Autodesk Fusion 360 part; units mm, degrees
(part 4 of 11)
  spline S51 degree 5 poles (-18.4507, -20.1557) (-18.4538, -20.1562) (-18.4598, -20.1573) (-18.469, -20.1589) (-18.4811, -20.161) (-18.4962, -20.1638) (-18.5113, -20.1666) (-18.5264, -20.1695) (-18.5414, -20.1724) (-18.5564, -20.1754) (-18.5713, -20.1785) (-18.5862, -20.1816) (-18.6011, -20.1848) (-18.6159, -20.1881) (-18.6307, -20.1914) (-18.6455, -20.1948) (-18.6602, -20.1983) (-18.6749, -20.2018) (-18.6895, -20.2054) (-18.7041, -20.209) (-18.7186, -20.2127) (-18.7332, -20.2165) (-18.7476, -20.2203) (-18.762, -20.2242) (-18.7764, -20.2282) (-18.7908, -20.2323) (-18.805, -20.2364) (-18.8193, -20.2406) (-18.8335, -20.2448) (-18.8476, -20.2491) (-18.8617, -20.2535) (-18.8758, -20.2579) (-18.8898, -20.2625) (-18.9038, -20.267) (-18.9177, -20.2717) (-18.9315, -20.2764) (-18.9453, -20.2812) (-18.9591, -20.2861) (-18.9728, -20.2911) (-18.9865, -20.2961) (-19.0001, -20.3012) (-19.0136, -20.3063) (-19.0271, -20.3116) (-19.0405, -20.3169) (-19.0539, -20.3223) (-19.0672, -20.3278) (-19.0805, -20.3333) (-19.0937, -20.3389) (-19.1068, -20.3447) (-19.1199, -20.3504) (-19.1329, -20.3563) (-19.1458, -20.3623) (-19.1587, -20.3683) (-19.1715, -20.3745) (-19.1842, -20.3807) (-19.1968, -20.387) (-19.2094, -20.3934) (-19.2219, -20.3999) (-19.2344, -20.4065) (-19.2468, -20.4131) (-19.259, -20.4199) (-19.2712, -20.4268) (-19.2832, -20.4339) (-19.2952, -20.4411) (-19.307, -20.4484) (-19.3187, -20.4558) (-19.3304, -20.4633) (-19.342, -20.4709) (-19.3535, -20.4785) (-19.3649, -20.4864) (-19.376, -20.4945) (-19.3846, -20.5013) (-19.3909, -20.5066) (-19.395, -20.5103) (-19.397, -20.5122) knots -1 -1 -1 -1 -1 -1 -0.98571429 -0.97142857 -0.95714286 -0.94285714 -0.92857143 -0.91428571 -0.9 -0.88571429 -0.87142857 -0.85714286 -0.84285714 -0.82857143 -0.81428571 -0.8 -0.78571429 -0.77142857 -0.75714286 -0.74285714 -0.72857143 -0.71428571 -0.7 -0.68571429 -0.67142857 -0.65714286 -0.64285714 -0.62857143 -0.61428571 -0.6 -0.58571429 -0.57142857 -0.55714286 -0.54285714 -0.52857143 -0.51428571 -0.5 -0.48571429 -0.47142857 -0.45714286 -0.44285714 -0.42857143 -0.41428571 -0.4 -0.38571429 -0.37142857 -0.35714286 -0.34285714 -0.32857143 -0.31428571 -0.3 -0.28571429 -0.27142857 -0.25714286 -0.24285714 -0.22857143 -0.21428571 -0.2 -0.18571429 -0.17142857 -0.15714286 -0.14285714 -0.12857143 -0.11428571 -0.1 -0.08571429 -0.07142857 -0.05714286 -0.04285714 -0.02857143 -0.01428571 0 0 0 0 0 0 construction
  line L57 (-19.397, -20.5122) -> (-19.4476, -20.5584) construction
  arc A104 (-19.7933, -20.5503) -> (-19.4476, -20.5584) centre (-19.6162, -20.3738) ccw construction
  arc A105 (-19.7933, -20.5503) -> (-19.8754, -20.4695) centre (-23.9648, -24.7074) ccw construction
  arc A106 (-19.8891, -20.1239) -> (-19.8754, -20.4695) centre (-19.7018, -20.2896) ccw construction
  line L58 (-19.8891, -20.1239) -> (-19.8437, -20.0726) construction
  spline S52 degree 5 poles (-19.8437, -20.0726) (-19.8419, -20.0705) (-19.8383, -20.0664) (-19.8331, -20.06) (-19.8264, -20.0513) (-19.8184, -20.0401) (-19.8108, -20.0286) (-19.8033, -20.017) (-19.7959, -20.0052) (-19.7887, -19.9934) (-19.7814, -19.9816) (-19.7743, -19.9696) (-19.7673, -19.9576) (-19.7604, -19.9454) (-19.7537, -19.9332) (-19.7471, -19.9208) (-19.7406, -19.9083) (-19.7343, -19.8958) (-19.728, -19.8831) (-19.7218, -19.8704) (-19.7157, -19.8577) (-19.7097, -19.8449) (-19.7037, -19.832) (-19.6979, -19.819) (-19.6921, -19.806) (-19.6865, -19.7929) (-19.6809, -19.7797) (-19.6754, -19.7665) (-19.67, -19.7532) (-19.6647, -19.7399) (-19.6594, -19.7265) (-19.6542, -19.713) (-19.6491, -19.6995) (-19.6441, -19.6859) (-19.6391, -19.6723) (-19.6343, -19.6586) (-19.6295, -19.6449) (-19.6247, -19.6311) (-19.6201, -19.6173) (-19.6155, -19.6034) (-19.611, -19.5895) (-19.6066, -19.5755) (-19.6022, -19.5614) (-19.5979, -19.5474) (-19.5937, -19.5332) (-19.5895, -19.5191) (-19.5855, -19.5048) (-19.5814, -19.4906) (-19.5775, -19.4763) (-19.5736, -19.4619) (-19.5698, -19.4475) (-19.5661, -19.4331) (-19.5624, -19.4186) (-19.5588, -19.4041) (-19.5552, -19.3895) (-19.5518, -19.3749) (-19.5483, -19.3603) (-19.545, -19.3456) (-19.5417, -19.3308) (-19.5385, -19.3161) (-19.5354, -19.3013) (-19.5323, -19.2864) (-19.5293, -19.2715) (-19.5263, -19.2566) (-19.5234, -19.2417) (-19.5206, -19.2267) (-19.5178, -19.2116) (-19.5151, -19.1966) (-19.5125, -19.1815) (-19.5099, -19.1663) (-19.5074, -19.1512) (-19.5054, -19.139) (-19.504, -19.1298) (-19.503, -19.1237) (-19.5026, -19.1207) knots 0 0 0 0 0 0 0.01428571 0.02857143 0.04285714 0.05714286 0.07142857 0.08571429 0.1 0.11428571 0.12857143 0.14285714 0.15714286 0.17142857 0.18571429 0.2 0.21428571 0.22857143 0.24285714 0.25714286 0.27142857 0.28571429 0.3 0.31428571 0.32857143 0.34285714 0.35714286 0.37142857 0.38571429 0.4 0.41428571 0.42857143 0.44285714 0.45714286 0.47142857 0.48571429 0.5 0.51428571 0.52857143 0.54285714 0.55714286 0.57142857 0.58571429 0.6 0.61428571 0.62857143 0.64285714 0.65714286 0.67142857 0.68571429 0.7 0.71428571 0.72857143 0.74285714 0.75714286 0.77142857 0.78571429 0.8 0.81428571 0.82857143 0.84285714 0.85714286 0.87142857 0.88571429 0.9 0.91428571 0.92857143 0.94285714 0.95714286 0.97142857 0.98571429 1 1 1 1 1 1 construction
  arc A107 (-19.5026, -19.1207) -> (-19.8167, -18.8837) centre (-23.9648, -24.7074) ccw construction
  spline S53 degree 5 poles (-19.8167, -18.8837) (-19.8195, -18.885) (-19.8251, -18.8875) (-19.8335, -18.8914) (-19.8446, -18.8967) (-19.8585, -18.9032) (-19.8724, -18.9099) (-19.8862, -18.9166) (-19.8999, -18.9233) (-19.9136, -18.9301) (-19.9273, -18.9369) (-19.9409, -18.9438) (-19.9544, -18.9507) (-19.9679, -18.9577) (-19.9813, -18.9647) (-19.9947, -18.9718) (-20.008, -18.979) (-20.0213, -18.9862) (-20.0345, -18.9934) (-20.0476, -19.0007) (-20.0607, -19.0081) (-20.0738, -19.0155) (-20.0867, -19.0229) (-20.0996, -19.0304) (-20.1125, -19.038) (-20.1253, -19.0456) (-20.138, -19.0533) (-20.1507, -19.061) (-20.1633, -19.0688) (-20.1759, -19.0766) (-20.1884, -19.0845) (-20.2008, -19.0924) (-20.2132, -19.1004) (-20.2255, -19.1085) (-20.2377, -19.1166) (-20.2499, -19.1247) (-20.2619, -19.1329) (-20.274, -19.1412) (-20.2859, -19.1495) (-20.2978, -19.1579) (-20.3096, -19.1663) (-20.3214, -19.1748) (-20.3331, -19.1834) (-20.3447, -19.192) (-20.3562, -19.2007) (-20.3676, -19.2094) (-20.379, -19.2182) (-20.3903, -19.2271) (-20.4015, -19.236) (-20.4126, -19.2449) (-20.4237, -19.254) (-20.4346, -19.2631) (-20.4455, -19.2723) (-20.4562, -19.2815) (-20.4669, -19.2908) (-20.4775, -19.3002) (-20.488, -19.3096) (-20.4984, -19.3191) (-20.5087, -19.3287) (-20.519, -19.3384) (-20.5291, -19.3481) (-20.539, -19.3579) (-20.5488, -19.3678) (-20.5585, -19.3779) (-20.568, -19.388) (-20.5774, -19.3982) (-20.5868, -19.4085) (-20.596, -19.4188) (-20.6052, -19.4291) (-20.6141, -19.4397) (-20.6227, -19.4504) (-20.6293, -19.4592) (-20.634, -19.466) (-20.637, -19.4706) (-20.6385, -19.4729) knots -1 -1 -1 -1 -1 -1 -0.98571429 -0.97142857 -0.95714286 -0.94285714 -0.92857143 -0.91428571 -0.9 -0.88571429 -0.87142857 -0.85714286 -0.84285714 -0.82857143 -0.81428571 -0.8 -0.78571429 -0.77142857 -0.75714286 -0.74285714 -0.72857143 -0.71428571 -0.7 -0.68571429 -0.67142857 -0.65714286 -0.64285714 -0.62857143 -0.61428571 -0.6 -0.58571429 -0.57142857 -0.55714286 -0.54285714 -0.52857143 -0.51428571 -0.5 -0.48571429 -0.47142857 -0.45714286 -0.44285714 -0.42857143 -0.41428571 -0.4 -0.38571429 -0.37142857 -0.35714286 -0.34285714 -0.32857143 -0.31428571 -0.3 -0.28571429 -0.27142857 -0.25714286 -0.24285714 -0.22857143 -0.21428571 -0.2 -0.18571429 -0.17142857 -0.15714286 -0.14285714 -0.12857143 -0.11428571 -0.1 -0.08571429 -0.07142857 -0.05714286 -0.04285714 -0.02857143 -0.01428571 0 0 0 0 0 0 construction
  line L59 (-20.6385, -19.4729) -> (-20.6753, -19.5306) construction
  arc A108 (-21.0114, -19.6123) -> (-20.6753, -19.5306) centre (-20.886, -19.396) ccw construction
  arc A109 (-21.0114, -19.6123) -> (-21.1116, -19.5555) centre (-23.9648, -24.7074) ccw construction
  arc A110 (-21.2143, -19.2252) -> (-21.1116, -19.5555) centre (-20.9905, -19.3368) ccw construction
  line L60 (-21.2143, -19.2252) -> (-21.1837, -19.1639) construction
  spline S54 degree 5 poles (-21.1837, -19.1639) (-21.1825, -19.1615) (-21.1801, -19.1565) (-21.1767, -19.149) (-21.1725, -19.1389) (-21.1677, -19.126) (-21.1633, -19.1129) (-21.1591, -19.0997) (-21.155, -19.0865) (-21.151, -19.0732) (-21.1471, -19.0599) (-21.1433, -19.0465) (-21.1397, -19.033) (-21.1362, -19.0195) (-21.1329, -19.0059) (-21.1297, -18.9923) (-21.1267, -18.9786) (-21.1238, -18.9648) (-21.121, -18.951) (-21.1183, -18.9371) (-21.1157, -18.9232) (-21.1132, -18.9093) (-21.1108, -18.8953) (-21.1085, -18.8812) (-21.1063, -18.8672) (-21.1042, -18.853) (-21.1022, -18.8389) (-21.1004, -18.8247) (-21.0986, -18.8105) (-21.0969, -18.7962) (-21.0953, -18.7819) (-21.0937, -18.7675) (-21.0923, -18.7532) (-21.091, -18.7388) (-21.0897, -18.7243) (-21.0885, -18.7098) (-21.0875, -18.6953) (-21.0865, -18.6808) (-21.0856, -18.6662) (-21.0847, -18.6516) (-21.084, -18.637) (-21.0833, -18.6224) (-21.0827, -18.6077) (-21.0822, -18.593) (-21.0818, -18.5782) (-21.0815, -18.5635) (-21.0812, -18.5487) (-21.081, -18.5339) (-21.0809, -18.519) (-21.0809, -18.5041) (-21.0809, -18.4892) (-21.081, -18.4743) (-21.0812, -18.4594) (-21.0815, -18.4444) (-21.0819, -18.4294) (-21.0823, -18.4144) (-21.0828, -18.3994) (-21.0833, -18.3843) (-21.084, -18.3693) (-21.0847, -18.3542) (-21.0855, -18.3391) (-21.0864, -18.3239) (-21.0873, -18.3088) (-21.0883, -18.2936) (-21.0894, -18.2784) (-21.0905, -18.2632) (-21.0917, -18.2479) (-21.093, -18.2327) (-21.0944, -18.2174) (-21.0958, -18.2021) (-21.0973, -18.1868) (-21.0986, -18.1746) (-21.0996, -18.1654) (-21.1002, -18.1592) (-21.1006, -18.1562) knots 0 0 0 0 0 0 0.01428571 0.02857143 0.04285714 0.05714286 0.07142857 0.08571429 0.1 0.11428571 0.12857143 0.14285714 0.15714286 0.17142857 0.18571429 0.2 0.21428571 0.22857143 0.24285714 0.25714286 0.27142857 0.28571429 0.3 0.31428571 0.32857143 0.34285714 0.35714286 0.37142857 0.38571429 0.4 0.41428571 0.42857143 0.44285714 0.45714286 0.47142857 0.48571429 0.5 0.51428571 0.52857143 0.54285714 0.55714286 0.57142857 0.58571429 0.6 0.61428571 0.62857143 0.64285714 0.65714286 0.67142857 0.68571429 0.7 0.71428571 0.72857143 0.74285714 0.75714286 0.77142857 0.78571429 0.8 0.81428571 0.82857143 0.84285714 0.85714286 0.87142857 0.88571429 0.9 0.91428571 0.92857143 0.94285714 0.95714286 0.97142857 0.98571429 1 1 1 1 1 1 construction
  arc A111 (-21.1006, -18.1562) -> (-21.4653, -18.0085) centre (-23.9648, -24.7074) ccw construction
  spline S55 degree 5 poles (-21.4653, -18.0085) (-21.4677, -18.0105) (-21.4724, -18.0144) (-21.4795, -18.0204) (-21.489, -18.0283) (-21.5007, -18.0382) (-21.5123, -18.0482) (-21.5239, -18.0583) (-21.5355, -18.0683) (-21.547, -18.0784) (-21.5584, -18.0885) (-21.5697, -18.0987) (-21.581, -18.1089) (-21.5922, -18.1192) (-21.6034, -18.1294) (-21.6144, -18.1397) (-21.6255, -18.1501) (-21.6364, -18.1605) (-21.6473, -18.1709) (-21.6581, -18.1813) (-21.6688, -18.1918) (-21.6795, -18.2024) (-21.6901, -18.2129) (-21.7006, -18.2235) (-21.7111, -18.2341) (-21.7215, -18.2448) (-21.7318, -18.2555) (-21.7421, -18.2663) (-21.7522, -18.277) (-21.7623, -18.2878) (-21.7724, -18.2987) (-21.7823, -18.3096) (-21.7922, -18.3205) (-21.802, -18.3314) (-21.8117, -18.3424) (-21.8213, -18.3535) (-21.8309, -18.3645) (-21.8404, -18.3756) (-21.8498, -18.3868) (-21.8591, -18.3979) (-21.8683, -18.4091) (-21.8775, -18.4204) (-21.8865, -18.4317) (-21.8955, -18.443) (-21.9044, -18.4543) (-21.9132, -18.4657) (-21.9219, -18.4772) (-21.9305, -18.4887) (-21.939, -18.5002) (-21.9474, -18.5117) (-21.9558, -18.5233) (-21.964, -18.5349) (-21.9721, -18.5466) (-21.9801, -18.5583) (-21.988, -18.5701) (-21.9958, -18.5819) (-22.0035, -18.5937) (-22.0111, -18.6056) (-22.0186, -18.6175) (-22.026, -18.6295) (-22.0332, -18.6415) (-22.0403, -18.6535) (-22.0472, -18.6657) (-22.0539, -18.6779) (-22.0605, -18.6901) (-22.067, -18.7024) (-22.0733, -18.7147) (-22.0796, -18.7271) (-22.0858, -18.7395) (-22.0917, -18.7519) (-22.0972, -18.7645) (-22.1013, -18.7747) (-22.104, -18.7825) (-22.1058, -18.7877) (-22.1066, -18.7903) knots -1 -1 -1 -1 -1 -1 -0.98571429 -0.97142857 -0.95714286 -0.94285714 -0.92857143 -0.91428571 -0.9 -0.88571429 -0.87142857 -0.85714286 -0.84285714 -0.82857143 -0.81428571 -0.8 -0.78571429 -0.77142857 -0.75714286 -0.74285714 -0.72857143 -0.71428571 -0.7 -0.68571429 -0.67142857 -0.65714286 -0.64285714 -0.62857143 -0.61428571 -0.6 -0.58571429 -0.57142857 -0.55714286 -0.54285714 -0.52857143 -0.51428571 -0.5 -0.48571429 -0.47142857 -0.45714286 -0.44285714 -0.42857143 -0.41428571 -0.4 -0.38571429 -0.37142857 -0.35714286 -0.34285714 -0.32857143 -0.31428571 -0.3 -0.28571429 -0.27142857 -0.25714286 -0.24285714 -0.22857143 -0.21428571 -0.2 -0.18571429 -0.17142857 -0.15714286 -0.14285714 -0.12857143 -0.11428571 -0.1 -0.08571429 -0.07142857 -0.05714286 -0.04285714 -0.02857143 -0.01428571 0 0 0 0 0 0 construction
  line L61 (-22.1066, -18.7903) -> (-22.1273, -18.8556) construction
  arc A112 (-22.4307, -19.0215) -> (-22.1273, -18.8556) centre (-22.3656, -18.7801) ccw construction
  arc A113 (-22.4307, -19.0215) -> (-22.5423, -18.9926) centre (-23.9648, -24.7074) ccw construction
  arc A114 (-22.7269, -18.7001) -> (-22.5423, -18.9926) centre (-22.4819, -18.75) ccw construction
  line L62 (-22.7269, -18.7001) -> (-22.7132, -18.633) construction
  spline S56 degree 5 poles (-22.7132, -18.633) (-22.7127, -18.6303) (-22.7116, -18.6249) (-22.7103, -18.6168) (-22.7089, -18.6059) (-22.7076, -18.5922) (-22.7067, -18.5784) (-22.7061, -18.5646) (-22.7056, -18.5508) (-22.7051, -18.5369) (-22.7048, -18.523) (-22.7046, -18.5091) (-22.7046, -18.4952) (-22.7047, -18.4812) (-22.705, -18.4673) (-22.7055, -18.4532) (-22.7061, -18.4392) (-22.7069, -18.4252) (-22.7078, -18.4111) (-22.7087, -18.397) (-22.7098, -18.3829) (-22.711, -18.3688) (-22.7123, -18.3546) (-22.7137, -18.3405) (-22.7153, -18.3263) (-22.7169, -18.3122) (-22.7187, -18.298) (-22.7205, -18.2838) (-22.7225, -18.2696) (-22.7245, -18.2553) (-22.7267, -18.2411) (-22.7289, -18.2269) (-22.7312, -18.2126) (-22.7337, -18.1983) (-22.7362, -18.1841) (-22.7388, -18.1698) (-22.7415, -18.1555) (-22.7443, -18.1412) (-22.7472, -18.1269) (-22.7502, -18.1126) (-22.7533, -18.0983) (-22.7564, -18.0839) (-22.7597, -18.0696) (-22.763, -18.0553) (-22.7664, -18.0409) (-22.7699, -18.0266) (-22.7735, -18.0122) (-22.7771, -17.9978) (-22.7808, -17.9835) (-22.7847, -17.9691) (-22.7886, -17.9547) (-22.7925, -17.9404) (-22.7966, -17.926) (-22.8007, -17.9116) (-22.8049, -17.8972) (-22.8092, -17.8828) (-22.8136, -17.8684) (-22.8181, -17.854) (-22.8226, -17.8396) (-22.8272, -17.8252) (-22.8319, -17.8108) (-22.8366, -17.7964) (-22.8414, -17.782) (-22.8463, -17.7676) (-22.8513, -17.7532) (-22.8563, -17.7389) (-22.8615, -17.7245) (-22.8667, -17.7101) (-22.8719, -17.6957) (-22.8773, -17.6813) (-22.8827, -17.6669) (-22.8871, -17.6553) (-22.8904, -17.6467) (-22.8926, -17.6409) (-22.8937, -17.6381) knots 0 0 0 0 0 0 0.01428571 0.02857143 0.04285714 0.05714286 0.07142857 0.08571429 0.1 0.11428571 0.12857143 0.14285714 0.15714286 0.17142857 0.18571429 0.2 0.21428571 0.22857143 0.24285714 0.25714286 0.27142857 0.28571429 0.3 0.31428571 0.32857143 0.34285714 0.35714286 0.37142857 0.38571429 0.4 0.41428571 0.42857143 0.44285714 0.45714286 0.47142857 0.48571429 0.5 0.51428571 0.52857143 0.54285714 0.55714286 0.57142857 0.58571429 0.6 0.61428571 0.62857143 0.64285714 0.65714286 0.67142857 0.68571429 0.7 0.71428571 0.72857143 0.74285714 0.75714286 0.77142857 0.78571429 0.8 0.81428571 0.82857143 0.84285714 0.85714286 0.87142857 0.88571429 0.9 0.91428571 0.92857143 0.94285714 0.95714286 0.97142857 0.98571429 1 1 1 1 1 1 construction
  arc A115 (-22.8937, -17.6381) -> (-23.2843, -17.5899) centre (-23.9648, -24.7074) ccw construction
  spline S57 degree 5 poles (-23.2843, -17.5899) (-23.2861, -17.5924) (-23.2896, -17.5974) (-23.2949, -17.605) (-23.302, -17.6151) (-23.3107, -17.6277) (-23.3194, -17.6404) (-23.328, -17.6531) (-23.3366, -17.6658) (-23.345, -17.6785) (-23.3534, -17.6913) (-23.3618, -17.704) (-23.37, -17.7168) (-23.3782, -17.7296) (-23.3863, -17.7424) (-23.3944, -17.7552) (-23.4023, -17.7681) (-23.4102, -17.7809) (-23.418, -17.7938) (-23.4258, -17.8067) (-23.4334, -17.8196) (-23.441, -17.8325) (-23.4485, -17.8455) (-23.456, -17.8584) (-23.4633, -17.8714) (-23.4706, -17.8844) (-23.4778, -17.8974) (-23.4849, -17.9105) (-23.4919, -17.9235) (-23.4989, -17.9366) (-23.5058, -17.9496) (-23.5126, -17.9627) (-23.5193, -17.9758) (-23.5259, -17.9889) (-23.5324, -18.0021) (-23.5389, -18.0152) (-23.5453, -18.0284) (-23.5515, -18.0415) (-23.5577, -18.0547) (-23.5638, -18.0679) (-23.5699, -18.0811) (-23.5758, -18.0944) (-23.5816, -18.1076) (-23.5873, -18.1209) (-23.593, -18.1341) (-23.5985, -18.1474) (-23.604, -18.1607) (-23.6093, -18.174) (-23.6146, -18.1874) (-23.6197, -18.2007) (-23.6248, -18.214) (-23.6297, -18.2274) (-23.6345, -18.2408) (-23.6392, -18.2542) (-23.6438, -18.2676) (-23.6483, -18.281) (-23.6527, -18.2944) (-23.6569, -18.3079) (-23.6611, -18.3213) (-23.6651, -18.3348) (-23.669, -18.3482) (-23.6727, -18.3617) (-23.6762, -18.3752) (-23.6796, -18.3888) (-23.6828, -18.4023) (-23.6858, -18.4158) (-23.6888, -18.4294) (-23.6917, -18.4429) (-23.6944, -18.4565) (-23.6969, -18.4701) (-23.699, -18.4837) (-23.7002, -18.4946) (-23.7009, -18.5028) (-23.7012, -18.5083) (-23.7014, -18.511) knots -1 -1 -1 -1 -1 -1 -0.98571429 -0.97142857 -0.95714286 -0.94285714 -0.92857143 -0.91428571 -0.9 -0.88571429 -0.87142857 -0.85714286 -0.84285714 -0.82857143 -0.81428571 -0.8 -0.78571429 -0.77142857 -0.75714286 -0.74285714 -0.72857143 -0.71428571 -0.7 -0.68571429 -0.67142857 -0.65714286 -0.64285714 -0.62857143 -0.61428571 -0.6 -0.58571429 -0.57142857 -0.55714286 -0.54285714 -0.52857143 -0.51428571 -0.5 -0.48571429 -0.47142857 -0.45714286 -0.44285714 -0.42857143 -0.41428571 -0.4 -0.38571429 -0.37142857 -0.35714286 -0.34285714 -0.32857143 -0.31428571 -0.3 -0.28571429 -0.27142857 -0.25714286 -0.24285714 -0.22857143 -0.21428571 -0.2 -0.18571429 -0.17142857 -0.15714286 -0.14285714 -0.12857143 -0.11428571 -0.1 -0.08571429 -0.07142857 -0.05714286 -0.04285714 -0.02857143 -0.01428571 0 0 0 0 0 0 construction
  line L63 (-23.7014, -18.511) -> (-23.7044, -18.5794) construction
  arc A116 (-23.9546, -18.8182) -> (-23.7044, -18.5794) centre (-23.9542, -18.5682) ccw construction
  arc A117 (-23.9546, -18.8182) -> (-24.0699, -18.8191) centre (-23.9648, -24.7074) ccw construction
  arc A118 (-24.3238, -18.5844) -> (-24.0699, -18.8191) centre (-24.0743, -18.5692) ccw construction
  line L64 (-24.3238, -18.5844) -> (-24.328, -18.5161) construction
  spline S58 degree 5 poles (-24.328, -18.5161) (-24.3282, -18.5133) (-24.3286, -18.5079) (-24.3294, -18.4997) (-24.3308, -18.4888) (-24.3332, -18.4752) (-24.3359, -18.4617) (-24.3388, -18.4482) (-24.3419, -18.4347) (-24.3451, -18.4212) (-24.3484, -18.4077) (-24.3518, -18.3942) (-24.3553, -18.3807) (-24.3591, -18.3673) (-24.363, -18.3538) (-24.3671, -18.3404) (-24.3713, -18.327) (-24.3757, -18.3137) (-24.3802, -18.3003) (-24.3848, -18.2869) (-24.3895, -18.2736) (-24.3943, -18.2603) (-24.3992, -18.247) (-24.4042, -18.2337) (-24.4094, -18.2204) (-24.4146, -18.2071) (-24.42, -18.1939) (-24.4255, -18.1806) (-24.431, -18.1674) (-24.4367, -18.1542) (-24.4425, -18.141) (-24.4483, -18.1278) (-24.4543, -18.1147) (-24.4603, -18.1015) (-24.4664, -18.0884) (-24.4727, -18.0753) (-24.479, -18.0621) (-24.4854, -18.0491) (-24.4919, -18.036) (-24.4985, -18.0229) (-24.5051, -18.0099) (-24.5119, -17.9969) (-24.5187, -17.9839) (-24.5256, -17.9709) (-24.5326, -17.9579) (-24.5397, -17.9449) (-24.5469, -17.932) (-24.5541, -17.9191) (-24.5615, -17.9062) (-24.5689, -17.8933) (-24.5764, -17.8804) (-24.5839, -17.8675) (-24.5916, -17.8547) (-24.5993, -17.8419) (-24.6071, -17.8291) (-24.6149, -17.8163) (-24.6229, -17.8035) (-24.6309, -17.7908) (-24.639, -17.778) (-24.6472, -17.7653) (-24.6554, -17.7526) (-24.6637, -17.7399) (-24.6721, -17.7273) (-24.6806, -17.7146) (-24.6891, -17.702) (-24.6977, -17.6894) (-24.7064, -17.6768) (-24.7151, -17.6643) (-24.7239, -17.6517) (-24.7328, -17.6392) (-24.7418, -17.6267) (-24.749, -17.6167) (-24.7544, -17.6092) (-24.7581, -17.6042) (-24.7599, -17.6017) knots 0 0 0 0 0 0 0.01428571 0.02857143 0.04285714 0.05714286 0.07142857 0.08571429 0.1 0.11428571 0.12857143 0.14285714 0.15714286 0.17142857 0.18571429 0.2 0.21428571 0.22857143 0.24285714 0.25714286 0.27142857 0.28571429 0.3 0.31428571 0.32857143 0.34285714 0.35714286 0.37142857 0.38571429 0.4 0.41428571 0.42857143 0.44285714 0.45714286 0.47142857 0.48571429 0.5 0.51428571 0.52857143 0.54285714 0.55714286 0.57142857 0.58571429 0.6 0.61428571 0.62857143 0.64285714 0.65714286 0.67142857 0.68571429 0.7 0.71428571 0.72857143 0.74285714 0.75714286 0.77142857 0.78571429 0.8 0.81428571 0.82857143 0.84285714 0.85714286 0.87142857 0.88571429 0.9 0.91428571 0.92857143 0.94285714 0.95714286 0.97142857 0.98571429 1 1 1 1 1 1 construction
  arc A119 (-24.7599, -17.6017) -> (-25.1496, -17.6563) centre (-23.9648, -24.7074) ccw construction
  spline S59 degree 5 poles (-25.1496, -17.6563) (-25.1507, -17.6591) (-25.1528, -17.6649) (-25.156, -17.6736) (-25.1602, -17.6852) (-25.1654, -17.6997) (-25.1705, -17.7142) (-25.1755, -17.7287) (-25.1805, -17.7431) (-25.1854, -17.7576) (-25.1902, -17.7721) (-25.1949, -17.7866) (-25.1996, -17.8011) (-25.2042, -17.8155) (-25.2087, -17.83) (-25.2131, -17.8445) (-25.2175, -17.8589) (-25.2218, -17.8734) (-25.226, -17.8879) (-25.2302, -17.9023) (-25.2342, -17.9168) (-25.2382, -17.9312) (-25.2421, -17.9457) (-25.2459, -17.9601) (-25.2497, -17.9746) (-25.2533, -17.989) (-25.2569, -18.0034) (-25.2604, -18.0179) (-25.2639, -18.0323) (-25.2672, -18.0467) (-25.2704, -18.0611) (-25.2736, -18.0755) (-25.2767, -18.0899) (-25.2797, -18.1043) (-25.2826, -18.1186) (-25.2855, -18.133) (-25.2882, -18.1474) (-25.2909, -18.1617) (-25.2934, -18.1761) (-25.2959, -18.1904) (-25.2983, -18.2047) (-25.3006, -18.219) (-25.3028, -18.2333) (-25.3049, -18.2476) (-25.3069, -18.2619) (-25.3089, -18.2762) (-25.3107, -18.2904) (-25.3124, -18.3047) (-25.314, -18.3189) (-25.3156, -18.3331) (-25.317, -18.3473) (-25.3183, -18.3615) (-25.3195, -18.3757) (-25.3205, -18.3898) (-25.3215, -18.4039) (-25.3224, -18.4181) (-25.3231, -18.4322) (-25.3238, -18.4462) (-25.3243, -18.4603) (-25.3247, -18.4744) (-25.325, -18.4884) (-25.3251, -18.5024) (-25.325, -18.5163) (-25.3247, -18.5302) (-25.3242, -18.5441) (-25.3237, -18.558) (-25.3231, -18.5719) (-25.3223, -18.5857) (-25.3215, -18.5995) (-25.3203, -18.6133) (-25.3189, -18.6269) (-25.3173, -18.6378) (-25.3158, -18.6459) (-25.3147, -18.6513) (-25.3141, -18.654) knots -1 -1 -1 -1 -1 -1 -0.98571429 -0.97142857 -0.95714286 -0.94285714 -0.92857143 -0.91428571 -0.9 -0.88571429 -0.87142857 -0.85714286 -0.84285714 -0.82857143 -0.81428571 -0.8 -0.78571429 -0.77142857 -0.75714286 -0.74285714 -0.72857143 -0.71428571 -0.7 -0.68571429 -0.67142857 -0.65714286 -0.64285714 -0.62857143 -0.61428571 -0.6 -0.58571429 -0.57142857 -0.55714286 -0.54285714 -0.52857143 -0.51428571 -0.5 -0.48571429 -0.47142857 -0.45714286 -0.44285714 -0.42857143 -0.41428571 -0.4 -0.38571429 -0.37142857 -0.35714286 -0.34285714 -0.32857143 -0.31428571 -0.3 -0.28571429 -0.27142857 -0.25714286 -0.24285714 -0.22857143 -0.21428571 -0.2 -0.18571429 -0.17142857 -0.15714286 -0.14285714 -0.12857143 -0.11428571 -0.1 -0.08571429 -0.07142857 -0.05714286 -0.04285714 -0.02857143 -0.01428571 0 0 0 0 0 0 construction
  line L65 (-25.3141, -18.654) -> (-25.2993, -18.7209) construction
  arc A120 (-25.4792, -19.0162) -> (-25.2993, -18.7209) centre (-25.5435, -18.7747) ccw construction
  arc A121 (-25.4792, -19.0162) -> (-25.5903, -19.047) centre (-23.9648, -24.7074) ccw construction
  arc A122 (-25.8964, -18.886) -> (-25.5903, -19.047) centre (-25.6593, -18.8067) ccw construction
  line L66 (-25.8964, -18.886) -> (-25.9181, -18.8211) construction
  spline S60 degree 5 poles (-25.9181, -18.8211) (-25.919, -18.8185) (-25.9208, -18.8133) (-25.9237, -18.8055) (-25.9279, -18.7954) (-25.9336, -18.7829) (-25.9397, -18.7705) (-25.9461, -18.7582) (-25.9526, -18.746) (-25.9591, -18.7338) (-25.9658, -18.7216) (-25.9726, -18.7095) (-25.9795, -18.6974) (-25.9866, -18.6853) (-25.9938, -18.6734) (-26.0013, -18.6615) (-26.0088, -18.6497) (-26.0165, -18.6379) (-26.0243, -18.6261) (-26.0322, -18.6144) (-26.0402, -18.6027) (-26.0483, -18.5911) (-26.0565, -18.5795) (-26.0648, -18.568) (-26.0732, -18.5565) (-26.0817, -18.545) (-26.0903, -18.5336) (-26.099, -18.5223) (-26.1078, -18.5109) (-26.1167, -18.4996) (-26.1257, -18.4884) (-26.1348, -18.4772) (-26.1439, -18.466) (-26.1531, -18.4548) (-26.1625, -18.4437) (-26.1719, -18.4327) (-26.1814, -18.4217) (-26.191, -18.4107) (-26.2006, -18.3997) (-26.2103, -18.3888) (-26.2202, -18.378) (-26.23, -18.3671) (-26.24, -18.3563) (-26.2501, -18.3456) (-26.2602, -18.3349) (-26.2704, -18.3242) (-26.2807, -18.3135) (-26.291, -18.3029) (-26.3014, -18.2923) (-26.3119, -18.2818) (-26.3225, -18.2713) (-26.3331, -18.2609) (-26.3438, -18.2504) (-26.3546, -18.24) (-26.3654, -18.2297) (-26.3763, -18.2194) (-26.3873, -18.2091) (-26.3984, -18.1989) (-26.4095, -18.1886) (-26.4207, -18.1785) (-26.4319, -18.1684) (-26.4432, -18.1583) (-26.4546, -18.1482) (-26.466, -18.1382) (-26.4775, -18.1282) (-26.4891, -18.1182) (-26.5008, -18.1083) (-26.5125, -18.0985) (-26.5242, -18.0886) (-26.536, -18.0788) (-26.5479, -18.0691) (-26.5575, -18.0613) (-26.5647, -18.0555) (-26.5695, -18.0516) (-26.5719, -18.0497) knots 0 0 0 0 0 0 0.01428571 0.02857143 0.04285714 0.05714286 0.07142857 0.08571429 0.1 0.11428571 0.12857143 0.14285714 0.15714286 0.17142857 0.18571429 0.2 0.21428571 0.22857143 0.24285714 0.25714286 0.27142857 0.28571429 0.3 0.31428571 0.32857143 0.34285714 0.35714286 0.37142857 0.38571429 0.4 0.41428571 0.42857143 0.44285714 0.45714286 0.47142857 0.48571429 0.5 0.51428571 0.52857143 0.54285714 0.55714286 0.57142857 0.58571429 0.6 0.61428571 0.62857143 0.64285714 0.65714286 0.67142857 0.68571429 0.7 0.71428571 0.72857143 0.74285714 0.75714286 0.77142857 0.78571429 0.8 0.81428571 0.82857143 0.84285714 0.85714286 0.87142857 0.88571429 0.9 0.91428571 0.92857143 0.94285714 0.95714286 0.97142857 0.98571429 1 1 1 1 1 1 construction
  arc A123 (-26.5719, -18.0497) -> (-26.9342, -18.2032) centre (-23.9648, -24.7074) ccw construction
  spline S61 degree 5 poles (-26.9342, -18.2032) (-26.9345, -18.2063) (-26.9351, -18.2124) (-26.9359, -18.2216) (-26.9369, -18.2339) (-26.9382, -18.2492) (-26.9394, -18.2645) (-26.9405, -18.2798) (-26.9415, -18.2951) (-26.9425, -18.3103) (-26.9434, -18.3256) (-26.9443, -18.3408) (-26.945, -18.356) (-26.9457, -18.3712) (-26.9463, -18.3863) (-26.9469, -18.4014) (-26.9473, -18.4165) (-26.9477, -18.4316) (-26.9481, -18.4467) (-26.9483, -18.4617) (-26.9485, -18.4767) (-26.9486, -18.4917) (-26.9486, -18.5067) (-26.9486, -18.5216) (-26.9485, -18.5365) (-26.9483, -18.5514) (-26.948, -18.5663) (-26.9477, -18.5811) (-26.9472, -18.5959) (-26.9467, -18.6107) (-26.9462, -18.6255) (-26.9455, -18.6402) (-26.9448, -18.6549) (-26.9439, -18.6696) (-26.943, -18.6842) (-26.942, -18.6988) (-26.941, -18.7134) (-26.9398, -18.728) (-26.9386, -18.7425) (-26.9373, -18.757) (-26.9359, -18.7714) (-26.9344, -18.7859) (-26.9328, -18.8002) (-26.9312, -18.8146) (-26.9294, -18.8289) (-26.9276, -18.8432) (-26.9257, -18.8574) (-26.9236, -18.8716) (-26.9215, -18.8858) (-26.9193, -18.8999) (-26.917, -18.914) (-26.9146, -18.928) (-26.9121, -18.942) (-26.9095, -18.956) (-26.9067, -18.9699) (-26.9039, -18.9837) (-26.901, -18.9976) (-26.898, -19.0113) (-26.8948, -19.025) (-26.8916, -19.0387) (-26.8882, -19.0523) (-26.8847, -19.0659) (-26.881, -19.0793) (-26.8771, -19.0927) (-26.8731, -19.106) (-26.869, -19.1193) (-26.8648, -19.1325) (-26.8605, -19.1457) (-26.8561, -19.1588) (-26.8514, -19.1718) (-26.8465, -19.1846) (-26.8421, -19.1947) (-26.8386, -19.2021) (-26.8361, -19.207) (-26.8348, -19.2095) knots -1 -1 -1 -1 -1 -1 -0.98571429 -0.97142857 -0.95714286 -0.94285714 -0.92857143 -0.91428571 -0.9 -0.88571429 -0.87142857 -0.85714286 -0.84285714 -0.82857143 -0.81428571 -0.8 -0.78571429 -0.77142857 -0.75714286 -0.74285714 -0.72857143 -0.71428571 -0.7 -0.68571429 -0.67142857 -0.65714286 -0.64285714 -0.62857143 -0.61428571 -0.6 -0.58571429 -0.57142857 -0.55714286 -0.54285714 -0.52857143 -0.51428571 -0.5 -0.48571429 -0.47142857 -0.45714286 -0.44285714 -0.42857143 -0.41428571 -0.4 -0.38571429 -0.37142857 -0.35714286 -0.34285714 -0.32857143 -0.31428571 -0.3 -0.28571429 -0.27142857 -0.25714286 -0.24285714 -0.22857143 -0.21428571 -0.2 -0.18571429 -0.17142857 -0.15714286 -0.14285714 -0.12857143 -0.11428571 -0.1 -0.08571429 -0.07142857 -0.05714286 -0.04285714 -0.02857143 -0.01428571 0 0 0 0 0 0 construction
  line L67 (-26.8348, -19.2095) -> (-26.8033, -19.2703) construction
  arc A124 (-26.9006, -19.6021) -> (-26.8033, -19.2703) centre (-27.0252, -19.3854) ccw construction
  arc A125 (-26.9006, -19.6021) -> (-26.9999, -19.6606) centre (-23.9648, -24.7074) ccw construction
  arc A126 (-27.3372, -19.5843) -> (-26.9999, -19.6606) centre (-27.1287, -19.4463) ccw construction
  line L68 (-27.3372, -19.5843) -> (-27.375, -19.5272) construction
  spline S62 degree 5 poles (-27.375, -19.5272) (-27.3765, -19.5249) (-27.3796, -19.5203) (-27.3844, -19.5136) (-27.3911, -19.5049) (-27.3999, -19.4943) (-27.409, -19.484) (-27.4183, -19.4738) (-27.4278, -19.4636) (-27.4373, -19.4535) (-27.4468, -19.4435) (-27.4565, -19.4335) (-27.4663, -19.4236) (-27.4763, -19.4138) (-27.4864, -19.4042) (-27.4967, -19.3946) (-27.507, -19.3851) (-27.5175, -19.3757) (-27.5281, -19.3664) (-27.5387, -19.3571) (-27.5495, -19.3479) (-27.5603, -19.3388) (-27.5712, -19.3297) (-27.5822, -19.3207) (-27.5933, -19.3118) (-27.6045, -19.3029) (-27.6158, -19.2941) (-27.6271, -19.2854) (-27.6386, -19.2767) (-27.6501, -19.2681) (-27.6617, -19.2596) (-27.6733, -19.2511) (-27.6851, -19.2427) (-27.6969, -19.2343) (-27.7087, -19.226) (-27.7207, -19.2177) (-27.7327, -19.2095) (-27.7448, -19.2014) (-27.757, -19.1933) (-27.7692, -19.1853) (-27.7815, -19.1774) (-27.7938, -19.1695) (-27.8063, -19.1616) (-27.8188, -19.1538) (-27.8313, -19.1461) (-27.8439, -19.1384) (-27.8566, -19.1308) (-27.8693, -19.1232) (-27.8821, -19.1157) (-27.895, -19.1082) (-27.9079, -19.1008) (-27.9209, -19.0935) (-27.9339, -19.0862) (-27.947, -19.0789) (-27.9602, -19.0717) (-27.9734, -19.0646) (-27.9867, -19.0575) (-28, -19.0505) (-28.0134, -19.0435) (-28.0268, -19.0366) (-28.0403, -19.0297) (-28.0538, -19.0229) (-28.0674, -19.0161) (-28.0811, -19.0094) (-28.0948, -19.0027) (-28.1085, -18.9961) (-28.1223, -18.9896) (-28.1362, -18.983) (-28.1501, -18.9766) (-28.164, -18.9702) (-28.178, -18.9638) (-28.1893, -18.9588) (-28.1977, -18.955) (-28.2034, -18.9525) (-28.2062, -18.9513) knots 0 0 0 0 0 0 0.01428571 0.02857143 0.04285714 0.05714286 0.07142857 0.08571429 0.1 0.11428571 0.12857143 0.14285714 0.15714286 0.17142857 0.18571429 0.2 0.21428571 0.22857143 0.24285714 0.25714286 0.27142857 0.28571429 0.3 0.31428571 0.32857143 0.34285714 0.35714286 0.37142857 0.38571429 0.4 0.41428571 0.42857143 0.44285714 0.45714286 0.47142857 0.48571429 0.5 0.51428571 0.52857143 0.54285714 0.55714286 0.57142857 0.58571429 0.6 0.61428571 0.62857143 0.64285714 0.65714286 0.67142857 0.68571429 0.7 0.71428571 0.72857143 0.74285714 0.75714286 0.77142857 0.78571429 0.8 0.81428571 0.82857143 0.84285714 0.85714286 0.87142857 0.88571429 0.9 0.91428571 0.92857143 0.94285714 0.95714286 0.97142857 0.98571429 1 1 1 1 1 1 construction
  arc A127 (-28.2062, -18.9513) -> (-28.5164, -19.1934) centre (-23.9648, -24.7074) ccw construction
  spline S63 degree 5 poles (-28.5164, -19.1934) (-28.5159, -19.1964) (-28.5149, -19.2025) (-28.5133, -19.2116) (-28.5111, -19.2237) (-28.5084, -19.2389) (-28.5056, -19.254) (-28.5027, -19.269) (-28.4997, -19.284) (-28.4967, -19.299) (-28.4937, -19.314) (-28.4905, -19.3289) (-28.4873, -19.3437) (-28.4841, -19.3586) (-28.4807, -19.3734) (-28.4774, -19.3881) (-28.4739, -19.4028) (-28.4704, -19.4175) (-28.4668, -19.4321) (-28.4632, -19.4467) (-28.4594, -19.4613) (-28.4557, -19.4758) (-28.4518, -19.4903) (-28.4479, -19.5047) (-28.4439, -19.519) (-28.4399, -19.5334) (-28.4358, -19.5477) (-28.4316, -19.5619) (-28.4274, -19.5761) (-28.4231, -19.5903) (-28.4187, -19.6044) (-28.4142, -19.6184) (-28.4097, -19.6324) (-28.4051, -19.6464) (-28.4005, -19.6603) (-28.3957, -19.6742) (-28.3909, -19.688) (-28.3861, -19.7017) (-28.3811, -19.7154) (-28.3761, -19.7291) (-28.371, -19.7427) (-28.3658, -19.7562) (-28.3606, -19.7697) (-28.3553, -19.7831) (-28.3499, -19.7965) (-28.3444, -19.8098) (-28.3388, -19.8231) (-28.3332, -19.8363) (-28.3275, -19.8494) (-28.3217, -19.8625) (-28.3159, -19.8755) (-28.3099, -19.8884) (-28.3038, -19.9013) (-28.2977, -19.9141) (-28.2915, -19.9268) (-28.2851, -19.9395) (-28.2787, -19.9521) (-28.2723, -19.9646) (-28.2657, -19.977) (-28.259, -19.9894) (-28.2522, -20.0017) (-28.2453, -20.0138) (-28.2383, -20.0259) (-28.2311, -20.0378) (-28.2237, -20.0496) (-28.2163, -20.0614) (-28.2088, -20.073) (-28.2013, -20.0846) (-28.1936, -20.0962) (-28.1858, -20.1075) (-28.1777, -20.1186) (-28.1709, -20.1272) (-28.1655, -20.1335) (-28.1619, -20.1376) (-28.16, -20.1396) knots -1 -1 -1 -1 -1 -1 -0.98571429 -0.97142857 -0.95714286 -0.94285714 -0.92857143 -0.91428571 -0.9 -0.88571429 -0.87142857 -0.85714286 -0.84285714 -0.82857143 -0.81428571 -0.8 -0.78571429 -0.77142857 -0.75714286 -0.74285714 -0.72857143 -0.71428571 -0.7 -0.68571429 -0.67142857 -0.65714286 -0.64285714 -0.62857143 -0.61428571 -0.6 -0.58571429 -0.57142857 -0.55714286 -0.54285714 -0.52857143 -0.51428571 -0.5 -0.48571429 -0.47142857 -0.45714286 -0.44285714 -0.42857143 -0.41428571 -0.4 -0.38571429 -0.37142857 -0.35714286 -0.34285714 -0.32857143 -0.31428571 -0.3 -0.28571429 -0.27142857 -0.25714286 -0.24285714 -0.22857143 -0.21428571 -0.2 -0.18571429 -0.17142857 -0.15714286 -0.14285714 -0.12857143 -0.11428571 -0.1 -0.08571429 -0.07142857 -0.05714286 -0.04285714 -0.02857143 -0.01428571 0 0 0 0 0 0 construction
  line L69 (-28.16, -20.1396) -> (-28.1138, -20.1902) construction
  arc A128 (-28.1219, -20.5359) -> (-28.1138, -20.1902) centre (-28.2983, -20.3588) ccw construction
  arc A129 (-28.1219, -20.5359) -> (-28.2027, -20.6181) centre (-23.9648, -24.7074) ccw construction
  arc A130 (-28.5483, -20.6317) -> (-28.2027, -20.6181) centre (-28.3826, -20.4445) ccw construction
  line L70 (-28.5483, -20.6317) -> (-28.5996, -20.5863) construction
  spline S64 degree 5 poles (-28.5996, -20.5863) (-28.6016, -20.5845) (-28.6058, -20.5809) (-28.6121, -20.5757) (-28.6209, -20.569) (-28.6321, -20.5611) (-28.6436, -20.5534) (-28.6552, -20.5459) (-28.6669, -20.5386) (-28.6787, -20.5313) (-28.6906, -20.5241) (-28.7025, -20.5169) (-28.7146, -20.5099) (-28.7267, -20.5031) (-28.739, -20.4963) (-28.7514, -20.4897) (-28.7639, -20.4833) (-28.7764, -20.4769) (-28.789, -20.4706) (-28.8017, -20.4644) (-28.8145, -20.4583) (-28.8273, -20.4523) (-28.8402, -20.4464) (-28.8531, -20.4405) (-28.8662, -20.4348) (-28.8793, -20.4291) (-28.8924, -20.4235) (-28.9057, -20.418) (-28.9189, -20.4126) (-28.9323, -20.4073) (-28.9457, -20.402) (-28.9592, -20.3968) (-28.9727, -20.3917) (-28.9862, -20.3867) (-28.9999, -20.3818) (-29.0135, -20.3769) (-29.0273, -20.3721) (-29.0411, -20.3674) (-29.0549, -20.3627) (-29.0688, -20.3581) (-29.0827, -20.3536) (-29.0967, -20.3492) (-29.1107, -20.3448) (-29.1248, -20.3405) (-29.1389, -20.3363) (-29.1531, -20.3322) (-29.1673, -20.3281) (-29.1816, -20.3241) (-29.1959, -20.3201) (-29.2102, -20.3162) (-29.2246, -20.3124) (-29.2391, -20.3087) (-29.2536, -20.305) (-29.2681, -20.3014) (-29.2827, -20.2979) (-29.2973, -20.2944) (-29.3119, -20.291) (-29.3266, -20.2876) (-29.3413, -20.2844) (-29.3561, -20.2811) (-29.3709, -20.278) (-29.3857, -20.2749) (-29.4006, -20.2719) (-29.4155, -20.2689) (-29.4305, -20.266) (-29.4455, -20.2632) (-29.4605, -20.2604) (-29.4756, -20.2577) (-29.4907, -20.2551) (-29.5058, -20.2525) (-29.521, -20.25) (-29.5332, -20.2481) (-29.5423, -20.2466) (-29.5484, -20.2457) (-29.5515, -20.2452) knots 0 0 0 0 0 0 0.01428571 0.02857143 0.04285714 0.05714286 0.07142857 0.08571429 0.1 0.11428571 0.12857143 0.14285714 0.15714286 0.17142857 0.18571429 0.2 0.21428571 0.22857143 0.24285714 0.25714286 0.27142857 0.28571429 0.3 0.31428571 0.32857143 0.34285714 0.35714286 0.37142857 0.38571429 0.4 0.41428571 0.42857143 0.44285714 0.45714286 0.47142857 0.48571429 0.5 0.51428571 0.52857143 0.54285714 0.55714286 0.57142857 0.58571429 0.6 0.61428571 0.62857143 0.64285714 0.65714286 0.67142857 0.68571429 0.7 0.71428571 0.72857143 0.74285714 0.75714286 0.77142857 0.78571429 0.8 0.81428571 0.82857143 0.84285714 0.85714286 0.87142857 0.88571429 0.9 0.91428571 0.92857143 0.94285714 0.95714286 0.97142857 0.98571429 1 1 1 1 1 1 construction
  arc A131 (-29.5515, -20.2452) -> (-29.7885, -20.5593) centre (-23.9648, -24.7074) ccw construction
  spline S65 degree 5 poles (-29.7885, -20.5593) (-29.7872, -20.5621) (-29.7846, -20.5677) (-29.7807, -20.5761) (-29.7755, -20.5873) (-29.7689, -20.6012) (-29.7623, -20.615) (-29.7556, -20.6288) (-29.7489, -20.6426) (-29.7421, -20.6563) (-29.7353, -20.6699) (-29.7284, -20.6835) (-29.7214, -20.697) (-29.7145, -20.7105) (-29.7074, -20.7239) (-29.7003, -20.7373) (-29.6932, -20.7506) (-29.686, -20.7639) (-29.6787, -20.7771) (-29.6714, -20.7903) (-29.6641, -20.8033) (-29.6567, -20.8164) (-29.6492, -20.8294) (-29.6417, -20.8423) (-29.6342, -20.8551) (-29.6265, -20.8679) (-29.6189, -20.8807) (-29.6112, -20.8933) (-29.6034, -20.906) (-29.5956, -20.9185) (-29.5877, -20.931) (-29.5797, -20.9434) (-29.5717, -20.9558) (-29.5637, -20.9681) (-29.5556, -20.9803) (-29.5474, -20.9925) (-29.5392, -21.0046) (-29.531, -21.0166) (-29.5226, -21.0286) (-29.5143, -21.0405) (-29.5058, -21.0523) (-29.4973, -21.064) (-29.4888, -21.0757) (-29.4802, -21.0873) (-29.4715, -21.0988) (-29.4627, -21.1102) (-29.454, -21.1216) (-29.4451, -21.1329) (-29.4362, -21.1441) (-29.4272, -21.1552) (-29.4182, -21.1663) (-29.4091, -21.1772) (-29.3999, -21.1881) (-29.3907, -21.1989) (-29.3813, -21.2095) (-29.372, -21.2201) (-29.3625, -21.2306) (-29.353, -21.241) (-29.3435, -21.2514) (-29.3338, -21.2616) (-29.3241, -21.2717) (-29.3143, -21.2816) (-29.3043, -21.2914) (-29.2943, -21.3011) (-29.2841, -21.3106) (-29.2739, -21.32) (-29.2637, -21.3294) (-29.2534, -21.3387) (-29.243, -21.3478) (-29.2325, -21.3567) (-29.2218, -21.3654) (-29.213, -21.3719) (-29.2062, -21.3766) (-29.2016, -21.3796) (-29.1993, -21.3811) knots -1 -1 -1 -1 -1 -1 -0.98571429 -0.97142857 -0.95714286 -0.94285714 -0.92857143 -0.91428571 -0.9 -0.88571429 -0.87142857 -0.85714286 -0.84285714 -0.82857143 -0.81428571 -0.8 -0.78571429 -0.77142857 -0.75714286 -0.74285714 -0.72857143 -0.71428571 -0.7 -0.68571429 -0.67142857 -0.65714286 -0.64285714 -0.62857143 -0.61428571 -0.6 -0.58571429 -0.57142857 -0.55714286 -0.54285714 -0.52857143 -0.51428571 -0.5 -0.48571429 -0.47142857 -0.45714286 -0.44285714 -0.42857143 -0.41428571 -0.4 -0.38571429 -0.37142857 -0.35714286 -0.34285714 -0.32857143 -0.31428571 -0.3 -0.28571429 -0.27142857 -0.25714286 -0.24285714 -0.22857143 -0.21428571 -0.2 -0.18571429 -0.17142857 -0.15714286 -0.14285714 -0.12857143 -0.11428571 -0.1 -0.08571429 -0.07142857 -0.05714286 -0.04285714 -0.02857143 -0.01428571 0 0 0 0 0 0 construction
  line L71 (-29.1993, -21.3811) -> (-29.1416, -21.418) construction
  arc A132 (-29.0599, -21.754) -> (-29.1416, -21.418) centre (-29.2762, -21.6286) ccw construction
  arc A133 (-29.0599, -21.754) -> (-29.1167, -21.8543) centre (-23.9648, -24.7074) ccw construction
  arc A134 (-29.4469, -21.9569) -> (-29.1167, -21.8543) centre (-29.3354, -21.7332) ccw construction
  line L72 (-29.4469, -21.9569) -> (-29.5082, -21.9263) construction
  spline S66 degree 5 poles (-29.5082, -21.9263) (-29.5107, -21.9251) (-29.5156, -21.9227) (-29.5231, -21.9193) (-29.5333, -21.9151) (-29.5462, -21.9103) (-29.5593, -21.9059) (-29.5725, -21.9017) (-29.5857, -21.8976) (-29.599, -21.8936) (-29.6123, -21.8897) (-29.6257, -21.8859) (-29.6391, -21.8823) (-29.6526, -21.8788) (-29.6662, -21.8755) (-29.6799, -21.8723) (-29.6936, -21.8693) (-29.7074, -21.8664) (-29.7212, -21.8636) (-29.7351, -21.8609) (-29.749, -21.8583) (-29.7629, -21.8558) (-29.7769, -21.8534) (-29.7909, -21.8511) (-29.805, -21.8489) (-29.8191, -21.8468) (-29.8333, -21.8449) (-29.8475, -21.843) (-29.8617, -21.8412) (-29.876, -21.8395) (-29.8903, -21.8379) (-29.9046, -21.8364) (-29.919, -21.8349) (-29.9334, -21.8336) (-29.9478, -21.8323) (-29.9623, -21.8312) (-29.9768, -21.8301) (-29.9914, -21.8291) (-30.0059, -21.8282) (-30.0205, -21.8274) (-30.0352, -21.8266) (-30.0498, -21.8259) (-30.0645, -21.8254) (-30.0792, -21.8249) (-30.0939, -21.8244) (-30.1087, -21.8241) (-30.1235, -21.8238) (-30.1383, -21.8236) (-30.1532, -21.8235) (-30.168, -21.8235) (-30.1829, -21.8235) (-30.1978, -21.8237) (-30.2128, -21.8239) (-30.2277, -21.8241) (-30.2427, -21.8245) (-30.2577, -21.8249) (-30.2728, -21.8254) (-30.2878, -21.826) (-30.3029, -21.8266) (-30.318, -21.8273) (-30.3331, -21.8281) (-30.3482, -21.829) (-30.3634, -21.8299) (-30.3786, -21.8309) (-30.3938, -21.832) (-30.409, -21.8332) (-30.4242, -21.8344) (-30.4395, -21.8357) (-30.4547, -21.837) (-30.47, -21.8385) (-30.4853, -21.84) (-30.4976, -21.8412) (-30.5068, -21.8422) (-30.5129, -21.8428) (-30.516, -21.8432) knots 0 0 0 0 0 0 0.01428571 0.02857143 0.04285714 0.05714286 0.07142857 0.08571429 0.1 0.11428571 0.12857143 0.14285714 0.15714286 0.17142857 0.18571429 0.2 0.21428571 0.22857143 0.24285714 0.25714286 0.27142857 0.28571429 0.3 0.31428571 0.32857143 0.34285714 0.35714286 0.37142857 0.38571429 0.4 0.41428571 0.42857143 0.44285714 0.45714286 0.47142857 0.48571429 0.5 0.51428571 0.52857143 0.54285714 0.55714286 0.57142857 0.58571429 0.6 0.61428571 0.62857143 0.64285714 0.65714286 0.67142857 0.68571429 0.7 0.71428571 0.72857143 0.74285714 0.75714286 0.77142857 0.78571429 0.8 0.81428571 0.82857143 0.84285714 0.85714286 0.87142857 0.88571429 0.9 0.91428571 0.92857143 0.94285714 0.95714286 0.97142857 0.98571429 1 1 1 1 1 1 construction
  arc A135 (-30.516, -21.8432) -> (-30.6637, -22.2079) centre (-23.9648, -24.7074) ccw construction
  spline S67 degree 5 poles (-30.6637, -22.2079) (-30.6617, -22.2103) (-30.6577, -22.2151) (-30.6518, -22.2222) (-30.6439, -22.2316) (-30.6339, -22.2433) (-30.6239, -22.255) (-30.6139, -22.2666) (-30.6038, -22.2781) (-30.5938, -22.2896) (-30.5836, -22.301) (-30.5735, -22.3123) (-30.5632, -22.3236) (-30.553, -22.3348) (-30.5427, -22.346) (-30.5324, -22.3571) (-30.5221, -22.3681) (-30.5117, -22.379) (-30.5013, -22.3899) (-30.4908, -22.4007) (-30.4803, -22.4115) (-30.4698, -22.4221) (-30.4592, -22.4327) (-30.4487, -22.4433) (-30.438, -22.4537) (-30.4274, -22.4641) (-30.4166, -22.4745) (-30.4059, -22.4847) (-30.3951, -22.4949) (-30.3843, -22.505) (-30.3735, -22.515) (-30.3626, -22.5249) (-30.3517, -22.5348) (-30.3407, -22.5446) (-30.3297, -22.5543) (-30.3187, -22.564) (-30.3076, -22.5735) (-30.2965, -22.583) (-30.2854, -22.5924) (-30.2742, -22.6017) (-30.263, -22.6109) (-30.2518, -22.6201) (-30.2405, -22.6292) (-30.2292, -22.6381) (-30.2178, -22.647) (-30.2064, -22.6558) (-30.195, -22.6645) (-30.1835, -22.6731) (-30.172, -22.6816) (-30.1605, -22.6901) (-30.1489, -22.6984) (-30.1372, -22.7066) (-30.1256, -22.7147) (-30.1138, -22.7227) (-30.1021, -22.7306) (-30.0903, -22.7384) (-30.0784, -22.7461) (-30.0666, -22.7537) (-30.0547, -22.7612) (-30.0427, -22.7686) (-30.0307, -22.7758) (-30.0186, -22.7829) (-30.0065, -22.7898) (-29.9943, -22.7965) (-29.982, -22.8031) (-29.9697, -22.8096) (-29.9574, -22.816) (-29.9451, -22.8222) (-29.9327, -22.8284) (-29.9202, -22.8343) (-29.9076, -22.8398) (-29.8974, -22.8439) (-29.8897, -22.8467) (-29.8844, -22.8484) (-29.8818, -22.8492) knots -1 -1 -1 -1 -1 -1 -0.98571429 -0.97142857 -0.95714286 -0.94285714 -0.92857143 -0.91428571 -0.9 -0.88571429 -0.87142857 -0.85714286 -0.84285714 -0.82857143 -0.81428571 -0.8 -0.78571429 -0.77142857 -0.75714286 -0.74285714 -0.72857143 -0.71428571 -0.7 -0.68571429 -0.67142857 -0.65714286 -0.64285714 -0.62857143 -0.61428571 -0.6 -0.58571429 -0.57142857 -0.55714286 -0.54285714 -0.52857143 -0.51428571 -0.5 -0.48571429 -0.47142857 -0.45714286 -0.44285714 -0.42857143 -0.41428571 -0.4 -0.38571429 -0.37142857 -0.35714286 -0.34285714 -0.32857143 -0.31428571 -0.3 -0.28571429 -0.27142857 -0.25714286 -0.24285714 -0.22857143 -0.21428571 -0.2 -0.18571429 -0.17142857 -0.15714286 -0.14285714 -0.12857143 -0.11428571 -0.1 -0.08571429 -0.07142857 -0.05714286 -0.04285714 -0.02857143 -0.01428571 0 0 0 0 0 0 construction
  line L73 (-29.8818, -22.8492) -> (-29.8165, -22.8699) construction
  arc A136 (-29.6507, -23.1734) -> (-29.8165, -22.8699) centre (-29.892, -23.1082) ccw construction
  arc A137 (-29.6507, -23.1734) -> (-29.6796, -23.2849) centre (-23.9648, -24.7074) ccw construction
  arc A138 (-29.972, -23.4695) -> (-29.6796, -23.2849) centre (-29.9222, -23.2245) ccw construction
  line L74 (-29.972, -23.4695) -> (-30.0391, -23.4558) construction
  spline S68 degree 5 poles (-30.0391, -23.4558) (-30.0418, -23.4553) (-30.0472, -23.4543) (-30.0554, -23.4529) (-30.0663, -23.4515) (-30.08, -23.4502) (-30.0937, -23.4493) (-30.1075, -23.4487) (-30.1214, -23.4482) (-30.1352, -23.4478) (-30.1491, -23.4474) (-30.163, -23.4472) (-30.177, -23.4472) (-30.1909, -23.4473) (-30.2049, -23.4476) (-30.2189, -23.4481) (-30.233, -23.4487) (-30.247, -23.4495) (-30.2611, -23.4504) (-30.2752, -23.4514) (-30.2893, -23.4524) (-30.3034, -23.4536) (-30.3175, -23.4549) (-30.3317, -23.4564) (-30.3458, -23.4579) (-30.36, -23.4595) (-30.3742, -23.4613) (-30.3884, -23.4631) (-30.4026, -23.4651) (-30.4168, -23.4672) (-30.4311, -23.4693) (-30.4453, -23.4715) (-30.4596, -23.4739) (-30.4738, -23.4763) (-30.4881, -23.4788) (-30.5024, -23.4815) (-30.5167, -23.4842) (-30.531, -23.487) (-30.5453, -23.4899) (-30.5596, -23.4928) (-30.5739, -23.4959) (-30.5882, -23.4991) (-30.6026, -23.5023) (-30.6169, -23.5056) (-30.6313, -23.509) (-30.6456, -23.5125) (-30.66, -23.5161) (-30.6743, -23.5197) (-30.6887, -23.5235) (-30.7031, -23.5273) (-30.7174, -23.5312) (-30.7318, -23.5352) (-30.7462, -23.5392) (-30.7606, -23.5434) (-30.775, -23.5476) (-30.7893, -23.5519) (-30.8037, -23.5562) (-30.8181, -23.5607) (-30.8325, -23.5652) (-30.8469, -23.5698) (-30.8613, -23.5745) (-30.8757, -23.5792) (-30.8901, -23.5841) (-30.9045, -23.589) (-30.9189, -23.5939) (-30.9333, -23.599) (-30.9477, -23.6041) (-30.9621, -23.6093) (-30.9765, -23.6146) (-30.9909, -23.6199) (-31.0053, -23.6253) (-31.0168, -23.6297) (-31.0255, -23.633) (-31.0312, -23.6352) (-31.0341, -23.6364) knots 0 0 0 0 0 0 0.01428571 0.02857143 0.04285714 0.05714286 0.07142857 0.08571429 0.1 0.11428571 0.12857143 0.14285714 0.15714286 0.17142857 0.18571429 0.2 0.21428571 0.22857143 0.24285714 0.25714286 0.27142857 0.28571429 0.3 0.31428571 0.32857143 0.34285714 0.35714286 0.37142857 0.38571429 0.4 0.41428571 0.42857143 0.44285714 0.45714286 0.47142857 0.48571429 0.5 0.51428571 0.52857143 0.54285714 0.55714286 0.57142857 0.58571429 0.6 0.61428571 0.62857143 0.64285714 0.65714286 0.67142857 0.68571429 0.7 0.71428571 0.72857143 0.74285714 0.75714286 0.77142857 0.78571429 0.8 0.81428571 0.82857143 0.84285714 0.85714286 0.87142857 0.88571429 0.9 0.91428571 0.92857143 0.94285714 0.95714286 0.97142857 0.98571429 1 1 1 1 1 1 construction
  arc A139 (-31.0341, -23.6364) -> (-31.0823, -24.0269) centre (-23.9648, -24.7074) ccw construction
  spline S69 degree 5 poles (-31.0823, -24.0269) (-31.0798, -24.0287) (-31.0747, -24.0323) (-31.0672, -24.0376) (-31.0571, -24.0446) (-31.0444, -24.0534) (-31.0318, -24.0621) (-31.0191, -24.0707) (-31.0064, -24.0792) (-30.9936, -24.0877) (-30.9809, -24.0961) (-30.9682, -24.1044) (-30.9554, -24.1127) (-30.9426, -24.1208) (-30.9298, -24.129) (-30.9169, -24.137) (-30.9041, -24.1449) (-30.8912, -24.1528) (-30.8784, -24.1607) (-30.8655, -24.1684) (-30.8526, -24.1761) (-30.8396, -24.1836) (-30.8267, -24.1911) (-30.8137, -24.1986) (-30.8007, -24.2059) (-30.7877, -24.2132) (-30.7747, -24.2204) (-30.7617, -24.2275) (-30.7487, -24.2346) (-30.7356, -24.2415) (-30.7225, -24.2484) (-30.7095, -24.2552) (-30.6964, -24.2619) (-30.6832, -24.2685) (-30.6701, -24.2751) (-30.657, -24.2815) (-30.6438, -24.2879) (-30.6306, -24.2942) (-30.6174, -24.3004) (-30.6042, -24.3065) (-30.591, -24.3125) (-30.5778, -24.3184) (-30.5645, -24.3242) (-30.5513, -24.33) (-30.538, -24.3356) (-30.5247, -24.3412) (-30.5114, -24.3466) (-30.4981, -24.352) (-30.4848, -24.3572) (-30.4715, -24.3624) (-30.4581, -24.3674) (-30.4448, -24.3723) (-30.4314, -24.3772) (-30.418, -24.3819) (-30.4046, -24.3865) (-30.3912, -24.3909) (-30.3777, -24.3953) (-30.3643, -24.3996) (-30.3509, -24.4037) (-30.3374, -24.4078) (-30.3239, -24.4116) (-30.3104, -24.4153) (-30.2969, -24.4189) (-30.2834, -24.4222) (-30.2699, -24.4254) (-30.2563, -24.4285) (-30.2428, -24.4314) (-30.2292, -24.4343) (-30.2157, -24.437) (-30.2021, -24.4395) (-30.1885, -24.4416) (-30.1776, -24.4429) (-30.1694, -24.4435) (-30.1639, -24.4439) (-30.1611, -24.444) knots -1 -1 -1 -1 -1 -1 -0.98571429 -0.97142857 -0.95714286 -0.94285714 -0.92857143 -0.91428571 -0.9 -0.88571429 -0.87142857 -0.85714286 -0.84285714 -0.82857143 -0.81428571 -0.8 -0.78571429 -0.77142857 -0.75714286 -0.74285714 -0.72857143 -0.71428571 -0.7 -0.68571429 -0.67142857 -0.65714286 -0.64285714 -0.62857143 -0.61428571 -0.6 -0.58571429 -0.57142857 -0.55714286 -0.54285714 -0.52857143 -0.51428571 -0.5 -0.48571429 -0.47142857 -0.45714286 -0.44285714 -0.42857143 -0.41428571 -0.4 -0.38571429 -0.37142857 -0.35714286 -0.34285714 -0.32857143 -0.31428571 -0.3 -0.28571429 -0.27142857 -0.25714286 -0.24285714 -0.22857143 -0.21428571 -0.2 -0.18571429 -0.17142857 -0.15714286 -0.14285714 -0.12857143 -0.11428571 -0.1 -0.08571429 -0.07142857 -0.05714286 -0.04285714 -0.02857143 -0.01428571 0 0 0 0 0 0 construction
  line L75 (-30.1611, -24.444) -> (-30.0927, -24.4471) construction